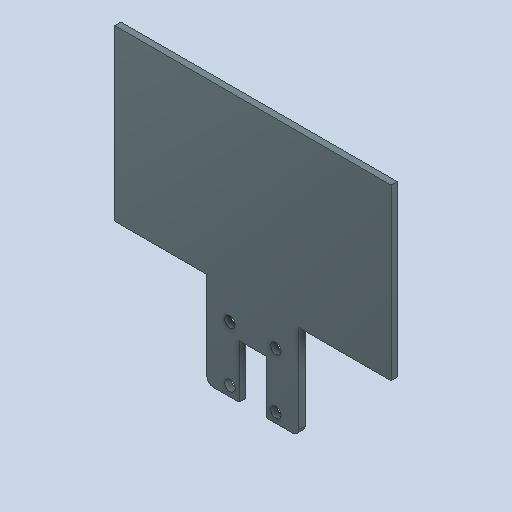
# Autodesk Inventor part: lead
Saved by Autodesk Inventor 2022 (Build 260153000, 153)
## iProperties
Created: 2022-12-25
Part Number: lead
Material: Lead
Document SubType Name: Modeling
Designer: Kamil
Mass: 143.662 g
Surface Area: 135.551 cm^2
Volume: 12.6686 cm^3
Density: 11.34 g/cm^3
Appearance: Lead
Author: Kamil
Autodesk Inventor part; units mm, degrees
ref_plane "YZ Plane" through (0, 0, 0) normal (1, 0, 0) x (0, 1, 0)
ref_plane "XZ Plane" through (0, 0, 0) normal (0, 1, 0) x (-1, 0, 0)
ref_plane "XY Plane" through (0, 0, 0) normal (0, 0, 1) x (1, 0, 0)
sketch "Sketch1" plane through (0, 0, 0) normal (0, 0, 1) x (1, 0, 0)
  line L0 (4.5, -29.1615) -> (4.5, -46.55) projected
  line L1 (4.5, -46.55) -> (13, -46.55) projected
  arc A0 (13, -46.55) -> (15, -44.55) centre (13, -44.55) ccw projected
  line L2 (15, -44.55) -> (15, -15.75) projected
  line L3 (15, -15.75) -> (45, -15.75) projected
  line L4 (45, 39.4571) -> (45, -15.75) projected
  line L5 (-45, -15.75) -> (-45, 39.4571) projected
  line L6 (-45, -15.75) -> (-15, -15.75) projected
  line L7 (-15, -15.75) -> (-15, -44.55) projected
  arc A1 (-15, -44.55) -> (-13, -46.55) centre (-13, -44.55) ccw projected
  line L8 (-13, -46.55) -> (-4.5, -46.55) projected
  line L9 (-4.5, -46.55) -> (-4.5, -29.1615) projected
  line L10 (-4.5, -29.1615) -> (4.5, -29.1615) projected
  circle A2 centre (7.5, -43.35) radius 1.75 projected
  circle A3 centre (7.5, -25.35) radius 1.75 projected
  circle A4 centre (-7.5, -25.35) radius 1.75 projected
  circle A5 centre (-7.5, -43.35) radius 1.75 projected
  line L11 (45, 39.4571) -> (-45, 39.4571) projected
  line L12 (-23.9404, 34.5074) -> (-20.8237, 34.5074) projected
  ellipse E0 centre (-19.8512, 32.8923) end of major axis (-19.8512, 35.0136) minor radius 1.5 (-18.8787, 34.5074) -> (-20.8237, 34.5074) ccw projected
  line L13 (-18.8787, 34.5074) -> (-15.7619, 34.5074) projected
  line L14 (-15.7619, 34.5074) -> (-15.7619, 27.8723) projected
  line L15 (-15.7619, 27.8723) -> (-23.9404, 27.8723) projected
  line L16 (-23.9404, 27.8723) -> (-23.9404, 34.5074) projected
  line L17 (15.7619, 34.5074) -> (18.8787, 34.5074) projected
  ellipse E1 centre (19.8512, 32.8923) end of major axis (19.8512, 35.0136) minor radius 1.5 (20.8237, 34.5074) -> (18.8787, 34.5074) ccw projected
  line L18 (20.8237, 34.5074) -> (23.9404, 34.5074) projected
  line L19 (23.9404, 34.5074) -> (23.9404, 27.8723) projected
  line L20 (23.9404, 27.8723) -> (15.7619, 27.8723) projected
  line L21 (15.7619, 27.8723) -> (15.7619, 34.5074) projected
  point P0 (0, 0)
  constraints: 2 other
extrude "Extrusion1" add sketch "Sketch1" along normal blind 2 contours L10 L9 L8 A1 L7 L6 L5 L11 L4 L3 L2 A0 L1 L0 | L12 E0 L13 L14 L15 L16 | L17 E1 L18 L19 L20 L21
body "Solid1"
